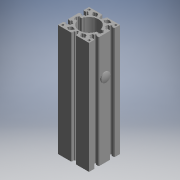
# Autodesk Inventor part: SLZ_63_Profil#_2871
Saved by Autodesk Inventor 2017.3 (Build 213256000, 256)
## iProperties
Part Number: SLZ_63_Profil#_2871
Material: Generic
Catalog Web Link: www.cadenas.de
Description: Profil Elektrozylinder SLZ 63-Control-Tec
Vendor: ROSEKRIEGER
Document SubType Name: Modeling
Designer: partserver
Manufacturer: ROSEKRIEGER
Mass: 785.447 g
Surface Area: 2909.04 cm^2
Volume: 785.447 cm^3
Density: 1 g/cm^3
Appearance: PSOLRGB-191-191-191
Category: PARTsolutions
Company: ROSEKRIEGER
Title: SLZ_63_Profil#_2871
Author: Cadenas PARTsolutions
Comments: Control-Tec
PSOL_IDENT_0: {$CADENAS_DATA\23d-libs\rose_krieger\linearkomponenten\pool_lineartechnik\_hubsaeule_zyliinder\elekt
PSOL_IDENT_1: rozylinder\elekzyl_slz63\parts\slz63_plfl_profil.prj},202 {VTYP=3D},{NB=SLZ_63_Profil#_2871},{LINA=S
PSOL_IDENT_2: LZ_63_Profil#_2871},{NN=Profil Elektrozylinder SLZ 63},{DATE=02.12.2020 11:16:24},{GEOMDATE=01.03.20
PSOL_IDENT_3: 17 09:52:29},{VERSION=},{LINEID=810},{WBVAR=},{WBNUMERIC=}  {NB=SLZ_63_Profil#_2871},{LINA=SLZ_63_Pr
PSOL_IDENT_4: ofil#_2871},{KT=DUMMY},{IDNR=},{CODE=TQ3},{ARTIKEL=Elektrozylinder },{TYPE=SLZ 63 Tr P PL},{BEST=SLZ
PSOL_IDENT_5: _63_Profil},{VARIANTE=PL},{SPINDEL=Tr 28x10},{SPINDELCODE=1.000},{SCHUTZARTVIS=IP54},{SCHUTZART=1},{
PSOL_IDENT_6: HUB1=0,[0:200]},{HUB2=200},{L1=287},{HINWEINBAUX=Hub + 274.5 mm},{DUMMYDURCH=10.000},{DUMMYLAENG=20.
PSOL_IDENT_7: 000},{HILFEHUB=105},{LAENDOPPROFIL=184.500},{RF=1.000},{GRUNDKOE=274.500},{XX=95.000},{A=100},{B=80}
PSOL_IDENT_8: ,{C=100},{D=125},{E=238},{F=40},{G=M16x1.5},{H=104},{K=125},{L=105},{M=48},{N=56.5},{O=86},{P=18.5},
PSOL_IDENT_9: {PPATH=sbl_lz70p_plfl.prj}
NB: SLZ_63_Profil#_2871
NN: Profil Elektrozylinder SLZ 63
NT: Control-Tec
NBSYN: $BEST.#_$L1.$SCHUTZART.
LINA: SLZ_63_Profil#_2871
CATALOG: RK Rose+Krieger
ARTIKEL: Elektrozylinder
TYPE: SLZ 63 Tr P PL
BEST: SLZ_63_Profil
SPINDEL: Tr 28x10
SPINDELCODE: 1
SCHUTZARTVIS: IP54
SCHUTZART: 1
HUB1: 0,[0:200]
HUB2: 200
L1: 287
HINWEINBAUX: Hub + 274.5 mm
DUMMYDURCH: 10
DUMMYLAENG: 20
HILFEHUB: 105
LAENDOPPROFIL: 184.5
RF: 1
GRUNDKOE: 274.5
XX: 95
A: 100
B: 80
C: 100
D: 125
E: 238
F: 40
G: M16x1.5
H: 104
K: 125
L: 105
M: 48
N: 56.5
O: 86
P: 18.5
SUPPLIER: ROSEKRIEGER
ARTICLENO: SLZ_63_Profil#_2871
BOMINFO: SLZ_63_Profil#_2871
CREATOR: CADENAS GmbH
Autodesk Inventor part; units mm, degrees
sketch "Sketch_1" plane through (0, 0, 0) normal (0, 0, 1) x (1, 0, 0)
  line L0 (-40, -26.375) -> (-40, -40)
  line L1 (-40, -40) -> (-6.3, -40)
  arc A0 (-6.3, -40) -> (-6.1, -39.8) centre (-6.3, -39.8) ccw
  line L2 (-6.1, -39.8) -> (-6.1, -38.7)
  arc A1 (-5.9, -38.5) -> (-6.1, -38.7) centre (-5.9, -38.7) ccw
  line L3 (-5.9, -38.5) -> (-5.3, -38.5)
  arc A2 (-5.3, -38.5) -> (-5.1, -38.3) centre (-5.3, -38.3) ccw
  line L4 (-5.1, -38.3) -> (-5.1, -33.2)
  arc A3 (-4.9, -33) -> (-5.1, -33.2) centre (-4.9, -33.2) ccw
  line L5 (-4.9, -33) -> (-2.95, -33)
  arc A4 (-2.95, -33) -> (-2.75, -32.8) centre (-2.95, -32.8) ccw
  line L6 (-2.75, -32.8) -> (-2.75, -28.6)
  arc A5 (-2.55, -28.4) -> (-2.75, -28.6) centre (-2.55, -28.6) ccw
  line L7 (-2.55, -28.4) -> (2.55, -28.4)
  arc A6 (2.75, -28.6) -> (2.55, -28.4) centre (2.55, -28.6) ccw
  line L8 (2.75, -28.6) -> (2.75, -32.8)
  arc A7 (2.75, -32.8) -> (2.95, -33) centre (2.95, -32.8) ccw
  line L9 (2.95, -33) -> (4.9, -33)
  arc A8 (5.1, -33.2) -> (4.9, -33) centre (4.9, -33.2) ccw
  line L10 (5.1, -33.2) -> (5.1, -38.3)
  arc A9 (5.1, -38.3) -> (5.3, -38.5) centre (5.3, -38.3) ccw
  line L11 (5.3, -38.5) -> (5.9, -38.5)
  arc A10 (6.1, -38.7) -> (5.9, -38.5) centre (5.9, -38.7) ccw
  line L12 (6.1, -38.7) -> (6.1, -39.8)
  arc A11 (6.1, -39.8) -> (6.3, -40) centre (6.3, -39.8) ccw
  line L13 (6.3, -40) -> (40, -40)
  line L14 (40, -40) -> (40, -26.375)
  arc A12 (40, -26.375) -> (39.7, -26.075) centre (39.7, -26.375) ccw
  line L15 (39.7, -26.075) -> (38.7, -26.075)
  arc A13 (38.5, -25.875) -> (38.7, -26.075) centre (38.7, -25.875) ccw
  line L16 (38.5, -25.875) -> (38.5, -25.4)
  arc A14 (38.5, -25.4) -> (38.2, -25.1) centre (38.2, -25.4) ccw
  line L17 (38.2, -25.1) -> (33.2, -25.1)
  arc A15 (33.2, -25.1) -> (33, -25.3) centre (33.2, -25.3) ccw
  line L18 (33, -25.3) -> (33, -27.55)
  arc A16 (32.8, -27.75) -> (33, -27.55) centre (32.8, -27.55) ccw
  line L19 (32.8, -27.75) -> (29.8328, -27.75)
  arc A17 (29.6914, -27.6914) -> (29.8328, -27.75) centre (29.8328, -27.55) ccw
  line L20 (29.6914, -27.6914) -> (28.5586, -26.5586)
  arc A18 (28.5, -26.4172) -> (28.5586, -26.5586) centre (28.7, -26.4172) ccw
  line L21 (28.5, -26.4172) -> (28.5, -24.45)
  arc A19 (28.5, -24.45) -> (28.3, -24.25) centre (28.3, -24.45) ccw
  line L22 (28.3, -24.25) -> (25, -24.25)
  arc A20 (24, -23.25) -> (25, -24.25) centre (25, -23.25) ccw
  line L23 (24, -23.25) -> (24, -20.3)
  arc A21 (24, -19.7) -> (24, -20.3) centre (24, -20) ccw
  line L24 (24, -19.7) -> (24, -16.75)
  arc A22 (25, -15.75) -> (24, -16.75) centre (25, -16.75) ccw
  line L25 (25, -15.75) -> (28.3, -15.75)
  arc A23 (28.3, -15.75) -> (28.5, -15.55) centre (28.3, -15.55) ccw
  line L26 (28.5, -15.55) -> (28.5, -13.5828)
  arc A24 (28.5586, -13.4414) -> (28.5, -13.5828) centre (28.7, -13.5828) ccw
  line L27 (28.5586, -13.4414) -> (29.6914, -12.3086)
  arc A25 (29.8328, -12.25) -> (29.6914, -12.3086) centre (29.8328, -12.45) ccw
  line L28 (29.8328, -12.25) -> (32.8, -12.25)
  arc A26 (33, -12.45) -> (32.8, -12.25) centre (32.8, -12.45) ccw
  line L29 (33, -12.45) -> (33, -14.7)
  arc A27 (33, -14.7) -> (33.2, -14.9) centre (33.2, -14.7) ccw
  line L30 (33.2, -14.9) -> (38.2, -14.9)
  arc A28 (38.2, -14.9) -> (38.5, -14.6) centre (38.2, -14.6) ccw
  line L31 (38.5, -14.6) -> (38.5, -14.125)
  arc A29 (38.7, -13.925) -> (38.5, -14.125) centre (38.7, -14.125) ccw
  line L32 (38.7, -13.925) -> (39.7, -13.925)
  arc A30 (39.7, -13.925) -> (40, -13.625) centre (39.7, -13.625) ccw
  line L33 (40, -13.625) -> (40, 13.625)
  arc A31 (40, 13.625) -> (39.7, 13.925) centre (39.7, 13.625) ccw
  line L34 (39.7, 13.925) -> (38.7, 13.925)
  arc A32 (38.5, 14.125) -> (38.7, 13.925) centre (38.7, 14.125) ccw
  line L35 (38.5, 14.125) -> (38.5, 14.6)
  arc A33 (38.5, 14.6) -> (38.2, 14.9) centre (38.2, 14.6) ccw
  line L36 (38.2, 14.9) -> (33.2, 14.9)
  arc A34 (33.2, 14.9) -> (33, 14.7) centre (33.2, 14.7) ccw
  line L37 (33, 14.7) -> (33, 12.45)
  arc A35 (32.8, 12.25) -> (33, 12.45) centre (32.8, 12.45) ccw
  line L38 (32.8, 12.25) -> (29.8328, 12.25)
  arc A36 (29.6914, 12.3086) -> (29.8328, 12.25) centre (29.8328, 12.45) ccw
  line L39 (29.6914, 12.3086) -> (28.5586, 13.4414)
  arc A37 (28.5, 13.5828) -> (28.5586, 13.4414) centre (28.7, 13.5828) ccw
  line L40 (28.5, 13.5828) -> (28.5, 15.55)
  arc A38 (28.5, 15.55) -> (28.3, 15.75) centre (28.3, 15.55) ccw
  line L41 (28.3, 15.75) -> (25, 15.75)
  arc A39 (24, 16.75) -> (25, 15.75) centre (25, 16.75) ccw
  line L42 (24, 16.75) -> (24, 19.7)
  arc A40 (24, 20.3) -> (24, 19.7) centre (24, 20) ccw
  line L43 (24, 20.3) -> (24, 23.25)
  arc A41 (25, 24.25) -> (24, 23.25) centre (25, 23.25) ccw
  line L44 (25, 24.25) -> (28.3, 24.25)
  arc A42 (28.3, 24.25) -> (28.5, 24.45) centre (28.3, 24.45) ccw
  line L45 (28.5, 24.45) -> (28.5, 26.4172)
  arc A43 (28.5586, 26.5586) -> (28.5, 26.4172) centre (28.7, 26.4172) ccw
  line L46 (28.5586, 26.5586) -> (29.6914, 27.6914)
  arc A44 (29.8328, 27.75) -> (29.6914, 27.6914) centre (29.8328, 27.55) ccw
  line L47 (29.8328, 27.75) -> (32.8, 27.75)
  arc A45 (33, 27.55) -> (32.8, 27.75) centre (32.8, 27.55) ccw
  line L48 (33, 27.55) -> (33, 25.3)
  arc A46 (33, 25.3) -> (33.2, 25.1) centre (33.2, 25.3) ccw
  line L49 (33.2, 25.1) -> (38.2, 25.1)
  arc A47 (38.2, 25.1) -> (38.5, 25.4) centre (38.2, 25.4) ccw
  line L50 (38.5, 25.4) -> (38.5, 25.875)
  arc A48 (38.7, 26.075) -> (38.5, 25.875) centre (38.7, 25.875) ccw
  line L51 (38.7, 26.075) -> (39.7, 26.075)
  arc A49 (39.7, 26.075) -> (40, 26.375) centre (39.7, 26.375) ccw
  line L52 (40, 26.375) -> (40, 40)
  line L53 (40, 40) -> (6.3, 40)
  arc A50 (6.3, 40) -> (6.1, 39.8) centre (6.3, 39.8) ccw
  line L54 (6.1, 39.8) -> (6.1, 38.7)
  arc A51 (5.9, 38.5) -> (6.1, 38.7) centre (5.9, 38.7) ccw
  line L55 (5.9, 38.5) -> (5.3, 38.5)
  arc A52 (5.3, 38.5) -> (5.1, 38.3) centre (5.3, 38.3) ccw
  line L56 (5.1, 38.3) -> (5.1, 33.2)
  arc A53 (4.9, 33) -> (5.1, 33.2) centre (4.9, 33.2) ccw
  line L57 (4.9, 33) -> (2.95, 33)
  arc A54 (2.95, 33) -> (2.75, 32.8) centre (2.95, 32.8) ccw
  line L58 (2.75, 32.8) -> (2.75, 28.6)
  arc A55 (2.55, 28.4) -> (2.75, 28.6) centre (2.55, 28.6) ccw
  line L59 (2.55, 28.4) -> (-2.55, 28.4)
  arc A56 (-2.75, 28.6) -> (-2.55, 28.4) centre (-2.55, 28.6) ccw
  line L60 (-2.75, 28.6) -> (-2.75, 32.8)
  arc A57 (-2.75, 32.8) -> (-2.95, 33) centre (-2.95, 32.8) ccw
  line L61 (-2.95, 33) -> (-4.9, 33)
  arc A58 (-5.1, 33.2) -> (-4.9, 33) centre (-4.9, 33.2) ccw
  line L62 (-5.1, 33.2) -> (-5.1, 38.3)
  arc A59 (-5.1, 38.3) -> (-5.3, 38.5) centre (-5.3, 38.3) ccw
  line L63 (-5.3, 38.5) -> (-5.9, 38.5)
  arc A60 (-6.1, 38.7) -> (-5.9, 38.5) centre (-5.9, 38.7) ccw
  line L64 (-6.1, 38.7) -> (-6.1, 39.8)
  arc A61 (-6.1, 39.8) -> (-6.3, 40) centre (-6.3, 39.8) ccw
  line L65 (-6.3, 40) -> (-40, 40)
  line L66 (-40, 40) -> (-40, 26.375)
  arc A62 (-40, 26.375) -> (-39.7, 26.075) centre (-39.7, 26.375) ccw
  line L67 (-39.7, 26.075) -> (-38.7, 26.075)
  arc A63 (-38.5, 25.875) -> (-38.7, 26.075) centre (-38.7, 25.875) ccw
  line L68 (-38.5, 25.875) -> (-38.5, 25.4)
  arc A64 (-38.5, 25.4) -> (-38.2, 25.1) centre (-38.2, 25.4) ccw
  line L69 (-38.2, 25.1) -> (-33.2, 25.1)
  arc A65 (-33.2, 25.1) -> (-33, 25.3) centre (-33.2, 25.3) ccw
  line L70 (-33, 25.3) -> (-33, 27.55)
  arc A66 (-32.8, 27.75) -> (-33, 27.55) centre (-32.8, 27.55) ccw
  line L71 (-32.8, 27.75) -> (-29.8328, 27.75)
  arc A67 (-29.6914, 27.6914) -> (-29.8328, 27.75) centre (-29.8328, 27.55) ccw
  line L72 (-29.6914, 27.6914) -> (-28.5586, 26.5586)
  arc A68 (-28.5, 26.4172) -> (-28.5586, 26.5586) centre (-28.7, 26.4172) ccw
  line L73 (-28.5, 26.4172) -> (-28.5, 24.45)
  arc A69 (-28.5, 24.45) -> (-28.3, 24.25) centre (-28.3, 24.45) ccw
  line L74 (-28.3, 24.25) -> (-25, 24.25)
  arc A70 (-24, 23.25) -> (-25, 24.25) centre (-25, 23.25) ccw
  line L75 (-24, 23.25) -> (-24, 20.3)
  arc A71 (-24, 19.7) -> (-24, 20.3) centre (-24, 20) ccw
  line L76 (-24, 19.7) -> (-24, 16.75)
  arc A72 (-25, 15.75) -> (-24, 16.75) centre (-25, 16.75) ccw
  line L77 (-25, 15.75) -> (-28.3, 15.75)
  arc A73 (-28.3, 15.75) -> (-28.5, 15.55) centre (-28.3, 15.55) ccw
  line L78 (-28.5, 15.55) -> (-28.5, 13.5828)
  arc A74 (-28.5586, 13.4414) -> (-28.5, 13.5828) centre (-28.7, 13.5828) ccw
  line L79 (-28.5586, 13.4414) -> (-29.6914, 12.3086)
  arc A75 (-29.8328, 12.25) -> (-29.6914, 12.3086) centre (-29.8328, 12.45) ccw
  line L80 (-29.8328, 12.25) -> (-32.8, 12.25)
  arc A76 (-33, 12.45) -> (-32.8, 12.25) centre (-32.8, 12.45) ccw
  line L81 (-33, 12.45) -> (-33, 14.7)
  arc A77 (-33, 14.7) -> (-33.2, 14.9) centre (-33.2, 14.7) ccw
  line L82 (-33.2, 14.9) -> (-38.2, 14.9)
  arc A78 (-38.2, 14.9) -> (-38.5, 14.6) centre (-38.2, 14.6) ccw
  line L83 (-38.5, 14.6) -> (-38.5, 14.125)
  arc A79 (-38.7, 13.925) -> (-38.5, 14.125) centre (-38.7, 14.125) ccw
  line L84 (-38.7, 13.925) -> (-39.7, 13.925)
  arc A80 (-39.7, 13.925) -> (-40, 13.625) centre (-39.7, 13.625) ccw
  line L85 (-40, 13.625) -> (-40, -13.625)
  arc A81 (-40, -13.625) -> (-39.7, -13.925) centre (-39.7, -13.625) ccw
  line L86 (-39.7, -13.925) -> (-38.7, -13.925)
  arc A82 (-38.5, -14.125) -> (-38.7, -13.925) centre (-38.7, -14.125) ccw
  line L87 (-38.5, -14.125) -> (-38.5, -14.6)
  arc A83 (-38.5, -14.6) -> (-38.2, -14.9) centre (-38.2, -14.6) ccw
  line L88 (-38.2, -14.9) -> (-33.2, -14.9)
  arc A84 (-33.2, -14.9) -> (-33, -14.7) centre (-33.2, -14.7) ccw
  line L89 (-33, -14.7) -> (-33, -12.45)
  arc A85 (-32.8, -12.25) -> (-33, -12.45) centre (-32.8, -12.45) ccw
  line L90 (-32.8, -12.25) -> (-29.8328, -12.25)
  arc A86 (-29.6914, -12.3086) -> (-29.8328, -12.25) centre (-29.8328, -12.45) ccw
  line L91 (-29.6914, -12.3086) -> (-28.5586, -13.4414)
  arc A87 (-28.5, -13.5828) -> (-28.5586, -13.4414) centre (-28.7, -13.5828) ccw
  line L92 (-28.5, -13.5828) -> (-28.5, -15.55)
  arc A88 (-28.5, -15.55) -> (-28.3, -15.75) centre (-28.3, -15.55) ccw
  line L93 (-28.3, -15.75) -> (-25, -15.75)
  arc A89 (-24, -16.75) -> (-25, -15.75) centre (-25, -16.75) ccw
  line L94 (-24, -16.75) -> (-24, -19.7)
  arc A90 (-24, -20.3) -> (-24, -19.7) centre (-24, -20) ccw
  line L95 (-24, -20.3) -> (-24, -23.25)
  arc A91 (-25, -24.25) -> (-24, -23.25) centre (-25, -23.25) ccw
  line L96 (-25, -24.25) -> (-28.3, -24.25)
  arc A92 (-28.3, -24.25) -> (-28.5, -24.45) centre (-28.3, -24.45) ccw
  line L97 (-28.5, -24.45) -> (-28.5, -26.4172)
  arc A93 (-28.5586, -26.5586) -> (-28.5, -26.4172) centre (-28.7, -26.4172) ccw
  line L98 (-28.5586, -26.5586) -> (-29.6914, -27.6914)
  arc A94 (-29.8328, -27.75) -> (-29.6914, -27.6914) centre (-29.8328, -27.55) ccw
  line L99 (-29.8328, -27.75) -> (-32.8, -27.75)
  arc A95 (-33, -27.55) -> (-32.8, -27.75) centre (-32.8, -27.55) ccw
  line L100 (-33, -27.55) -> (-33, -25.3)
  arc A96 (-33, -25.3) -> (-33.2, -25.1) centre (-33.2, -25.3) ccw
  line L101 (-33.2, -25.1) -> (-38.2, -25.1)
  arc A97 (-38.2, -25.1) -> (-38.5, -25.4) centre (-38.2, -25.4) ccw
  line L102 (-38.5, -25.4) -> (-38.5, -25.875)
  arc A98 (-38.7, -26.075) -> (-38.5, -25.875) centre (-38.7, -25.875) ccw
  line L103 (-38.7, -26.075) -> (-39.7, -26.075)
  arc A99 (-39.7, -26.075) -> (-40, -26.375) centre (-39.7, -26.375) ccw
  arc A100 (31.6024, 35.3468) -> (31.6024, 32.6532) centre (34, 34) ccw
  arc A101 (31.6024, 32.6532) -> (32.6532, 31.6024) centre (32.0555, 32.0555) ccw
  arc A102 (32.6532, 31.6024) -> (35.3468, 31.6024) centre (34, 34) ccw
  arc A103 (35.3468, 31.6024) -> (36.3976, 32.6532) centre (35.9445, 32.0555) ccw
  arc A104 (36.3976, 32.6532) -> (36.3976, 35.3468) centre (34, 34) ccw
  arc A105 (36.3976, 35.3468) -> (35.3468, 36.3976) centre (35.9445, 35.9445) ccw
  arc A106 (35.3468, 36.3976) -> (32.6532, 36.3976) centre (34, 34) ccw
  arc A107 (32.6532, 36.3976) -> (31.6024, 35.3468) centre (32.0555, 35.9445) ccw
  arc A108 (31.6024, -32.6532) -> (31.6024, -35.3468) centre (34, -34) ccw
  arc A109 (31.6024, -35.3468) -> (32.6532, -36.3976) centre (32.0555, -35.9445) ccw
  arc A110 (32.6532, -36.3976) -> (35.3468, -36.3976) centre (34, -34) ccw
  arc A111 (35.3468, -36.3976) -> (36.3976, -35.3468) centre (35.9445, -35.9445) ccw
  arc A112 (36.3976, -35.3468) -> (36.3976, -32.6532) centre (34, -34) ccw
  arc A113 (36.3976, -32.6532) -> (35.3468, -31.6024) centre (35.9445, -32.0555) ccw
  arc A114 (35.3468, -31.6024) -> (32.6532, -31.6024) centre (34, -34) ccw
  arc A115 (32.6532, -31.6024) -> (31.6024, -32.6532) centre (32.0555, -32.0555) ccw
  arc A116 (10.3501, 31.0384) -> (11.6966, 27.3389) centre (10.6907, 29.0676) ccw
  arc A117 (11.6966, 27.3389) -> (21.6499, 30.9616) centre (16, 31) ccw
  arc A118 (21.6499, 30.9616) -> (20.3034, 34.6611) centre (21.3093, 32.9324) ccw
  arc A119 (20.3034, 34.6611) -> (10.3501, 31.0384) centre (16, 31) ccw
  arc A120 (11.6966, -27.3389) -> (10.3501, -31.0384) centre (10.6907, -29.0676) ccw
  arc A121 (10.3501, -31.0384) -> (20.3034, -34.6611) centre (16, -31) ccw
  arc A122 (20.3034, -34.6611) -> (21.6499, -30.9616) centre (21.3093, -32.9324) ccw
  arc A123 (21.6499, -30.9616) -> (11.6966, -27.3389) centre (16, -31) ccw
  arc A124 (-21.6499, -30.9616) -> (-20.3034, -34.6611) centre (-21.3093, -32.9324) ccw
  arc A125 (-20.3034, -34.6611) -> (-10.3501, -31.0384) centre (-16, -31) ccw
  arc A126 (-10.3501, -31.0384) -> (-11.6966, -27.3389) centre (-10.6907, -29.0676) ccw
  arc A127 (-11.6966, -27.3389) -> (-21.6499, -30.9616) centre (-16, -31) ccw
  arc A128 (-20.3034, 34.6611) -> (-21.6499, 30.9616) centre (-21.3093, 32.9324) ccw
  arc A129 (-21.6499, 30.9616) -> (-11.6966, 27.3389) centre (-16, 31) ccw
  arc A130 (-11.6966, 27.3389) -> (-10.3501, 31.0384) centre (-10.6907, 29.0676) ccw
  arc A131 (-10.3501, 31.0384) -> (-20.3034, 34.6611) centre (-16, 31) ccw
  line L104 (-35, 1.95) -> (-35, -1.95)
  arc A132 (-35, -1.95) -> (-34.8, -2.15) centre (-34.8, -1.95) ccw
  line L105 (-34.8, -2.15) -> (-33.7, -2.15)
  arc A133 (-33.5, -2.35) -> (-33.7, -2.15) centre (-33.7, -2.35) ccw
  line L106 (-33.5, -2.35) -> (-33.5, -4.95)
  arc A134 (-33.5, -4.95) -> (-33.3, -5.15) centre (-33.3, -4.95) ccw
  line L107 (-33.3, -5.15) -> (-31.7, -5.15)
  arc A135 (-31.5, -5.35) -> (-31.7, -5.15) centre (-31.7, -5.35) ccw
  line L108 (-31.5, -5.35) -> (-31.5, -7.1)
  arc A136 (-31.5, -7.1) -> (-31.3, -7.3) centre (-31.3, -7.1) ccw
  line L109 (-31.3, -7.3) -> (-30, -7.3)
  arc A137 (-30, -7.3) -> (-29.8, -7.1) centre (-30, -7.1) ccw
  line L110 (-29.8, -7.1) -> (-29.8, -5.3)
  arc A138 (-29.6, -5.1) -> (-29.8, -5.3) centre (-29.6, -5.3) ccw
  line L111 (-29.6, -5.1) -> (-29.4, -5.1)
  arc A139 (-29.2, -5.3) -> (-29.4, -5.1) centre (-29.4, -5.3) ccw
  arc A140 (-29.2, -5.3) -> (-29, -5.5) centre (-29, -5.3) ccw
  line L112 (-29, -5.5) -> (-24.5469, -5.5)
  arc A141 (-24.3521, -5.6548) -> (-24.5469, -5.5) centre (-24.5469, -5.7) ccw
  arc A142 (-24.3521, -5.6548) -> (-23.4523, -8.6598) centre (0, 0) ccw
  arc A143 (-23.4551, -8.8056) -> (-23.4523, -8.6598) centre (-23.6399, -8.7291) ccw
  line L113 (-23.4551, -8.8056) -> (-23.91, -9.9038)
  line L114 (-23.91, -9.9038) -> (-22.8118, -10.3588)
  arc A144 (-22.7066, -10.4599) -> (-22.8118, -10.3588) centre (-22.8883, -10.5435) ccw
  arc A145 (-22.7066, -10.4599) -> (-10.4599, -22.7066) centre (0, 0) ccw
  arc A146 (-10.3588, -22.8118) -> (-10.4599, -22.7066) centre (-10.5435, -22.8883) ccw
  line L115 (-10.3588, -22.8118) -> (-9.9804, -23.7252)
  arc A147 (-9.9804, -23.7252) -> (-9.7191, -23.8335) centre (-9.7956, -23.6487) ccw
  line L116 (-9.7191, -23.8335) -> (-8.8056, -23.4551)
  arc A148 (-8.6598, -23.4523) -> (-8.8056, -23.4551) centre (-8.7291, -23.6399) ccw
  arc A149 (-8.6598, -23.4523) -> (8.6598, -23.4523) centre (0, 0) ccw
  arc A150 (8.8056, -23.4551) -> (8.6598, -23.4523) centre (8.7291, -23.6399) ccw
  line L117 (8.8056, -23.4551) -> (9.7191, -23.8335)
  arc A151 (9.7191, -23.8335) -> (9.9804, -23.7252) centre (9.7956, -23.6487) ccw
  line L118 (9.9804, -23.7252) -> (10.3588, -22.8118)
  arc A152 (10.4599, -22.7066) -> (10.3588, -22.8118) centre (10.5435, -22.8883) ccw
  arc A153 (10.4599, -22.7066) -> (22.7066, -10.4599) centre (0, 0) ccw
  arc A154 (22.8118, -10.3588) -> (22.7066, -10.4599) centre (22.8883, -10.5435) ccw
  line L119 (22.8118, -10.3588) -> (23.91, -9.9038)
  line L120 (23.91, -9.9038) -> (23.4551, -8.8056)
  arc A155 (23.4523, -8.6598) -> (23.4551, -8.8056) centre (23.6399, -8.7291) ccw
  arc A156 (23.4523, -8.6598) -> (24.3521, -5.6548) centre (0, 0) ccw
  arc A157 (24.5469, -5.5) -> (24.3521, -5.6548) centre (24.5469, -5.7) ccw
  line L121 (24.5469, -5.5) -> (29, -5.5)
  arc A158 (29, -5.5) -> (29.2, -5.3) centre (29, -5.3) ccw
  arc A159 (29.4, -5.1) -> (29.2, -5.3) centre (29.4, -5.3) ccw
  line L122 (29.4, -5.1) -> (29.6, -5.1)
  arc A160 (29.8, -5.3) -> (29.6, -5.1) centre (29.6, -5.3) ccw
  line L123 (29.8, -5.3) -> (29.8, -7.1)
  arc A161 (29.8, -7.1) -> (30, -7.3) centre (30, -7.1) ccw
  line L124 (30, -7.3) -> (31.3, -7.3)
  arc A162 (31.3, -7.3) -> (31.5, -7.1) centre (31.3, -7.1) ccw
  line L125 (31.5, -7.1) -> (31.5, -5.35)
  arc A163 (31.7, -5.15) -> (31.5, -5.35) centre (31.7, -5.35) ccw
  line L126 (31.7, -5.15) -> (33.3, -5.15)
  arc A164 (33.3, -5.15) -> (33.5, -4.95) centre (33.3, -4.95) ccw
  line L127 (33.5, -4.95) -> (33.5, -2.35)
  arc A165 (33.7, -2.15) -> (33.5, -2.35) centre (33.7, -2.35) ccw
  line L128 (33.7, -2.15) -> (34.8, -2.15)
  arc A166 (34.8, -2.15) -> (35, -1.95) centre (34.8, -1.95) ccw
  line L129 (35, -1.95) -> (35, 1.95)
  arc A167 (35, 1.95) -> (34.8, 2.15) centre (34.8, 1.95) ccw
  line L130 (34.8, 2.15) -> (33.7, 2.15)
  arc A168 (33.5, 2.35) -> (33.7, 2.15) centre (33.7, 2.35) ccw
  line L131 (33.5, 2.35) -> (33.5, 4.95)
  arc A169 (33.5, 4.95) -> (33.3, 5.15) centre (33.3, 4.95) ccw
  line L132 (33.3, 5.15) -> (31.7, 5.15)
  arc A170 (31.5, 5.35) -> (31.7, 5.15) centre (31.7, 5.35) ccw
  line L133 (31.5, 5.35) -> (31.5, 7.1)
  arc A171 (31.5, 7.1) -> (31.3, 7.3) centre (31.3, 7.1) ccw
  line L134 (31.3, 7.3) -> (30, 7.3)
  arc A172 (30, 7.3) -> (29.8, 7.1) centre (30, 7.1) ccw
  line L135 (29.8, 7.1) -> (29.8, 5.3)
  arc A173 (29.6, 5.1) -> (29.8, 5.3) centre (29.6, 5.3) ccw
  line L136 (29.6, 5.1) -> (29.4, 5.1)
  arc A174 (29.2, 5.3) -> (29.4, 5.1) centre (29.4, 5.3) ccw
  arc A175 (29.2, 5.3) -> (29, 5.5) centre (29, 5.3) ccw
  line L137 (29, 5.5) -> (24.5469, 5.5)
  arc A176 (24.3521, 5.6548) -> (24.5469, 5.5) centre (24.5469, 5.7) ccw
  arc A177 (24.3521, 5.6548) -> (23.4523, 8.6598) centre (0, 0) ccw
  arc A178 (23.4551, 8.8056) -> (23.4523, 8.6598) centre (23.6399, 8.7291) ccw
  line L138 (23.4551, 8.8056) -> (23.91, 9.9038)
  line L139 (23.91, 9.9038) -> (22.8118, 10.3588)
  arc A179 (22.7066, 10.4599) -> (22.8118, 10.3588) centre (22.8883, 10.5435) ccw
  arc A180 (22.7066, 10.4599) -> (10.4599, 22.7066) centre (0, 0) ccw
  arc A181 (10.3588, 22.8118) -> (10.4599, 22.7066) centre (10.5435, 22.8883) ccw
  line L140 (10.3588, 22.8118) -> (9.9804, 23.7252)
  arc A182 (9.9804, 23.7252) -> (9.7191, 23.8335) centre (9.7956, 23.6487) ccw
  line L141 (9.7191, 23.8335) -> (8.8056, 23.4551)
  arc A183 (8.6598, 23.4523) -> (8.8056, 23.4551) centre (8.7291, 23.6399) ccw
  arc A184 (8.6598, 23.4523) -> (-8.6598, 23.4523) centre (0, 0) ccw
  arc A185 (-8.8056, 23.4551) -> (-8.6598, 23.4523) centre (-8.7291, 23.6399) ccw
  line L142 (-8.8056, 23.4551) -> (-9.7191, 23.8335)
  arc A186 (-9.7191, 23.8335) -> (-9.9804, 23.7252) centre (-9.7956, 23.6487) ccw
  line L143 (-9.9804, 23.7252) -> (-10.3588, 22.8118)
  arc A187 (-10.4599, 22.7066) -> (-10.3588, 22.8118) centre (-10.5435, 22.8883) ccw
  arc A188 (-10.4599, 22.7066) -> (-22.7066, 10.4599) centre (0, 0) ccw
  arc A189 (-22.8118, 10.3588) -> (-22.7066, 10.4599) centre (-22.8883, 10.5435) ccw
  line L144 (-22.8118, 10.3588) -> (-23.91, 9.9038)
  line L145 (-23.91, 9.9038) -> (-23.4551, 8.8056)
  arc A190 (-23.4523, 8.6598) -> (-23.4551, 8.8056) centre (-23.6399, 8.7291) ccw
  arc A191 (-23.4523, 8.6598) -> (-24.3521, 5.6548) centre (0, 0) ccw
  arc A192 (-24.5469, 5.5) -> (-24.3521, 5.6548) centre (-24.5469, 5.7) ccw
  line L146 (-24.5469, 5.5) -> (-29, 5.5)
  arc A193 (-29, 5.5) -> (-29.2, 5.3) centre (-29, 5.3) ccw
  arc A194 (-29.4, 5.1) -> (-29.2, 5.3) centre (-29.4, 5.3) ccw
  line L147 (-29.4, 5.1) -> (-29.6, 5.1)
  arc A195 (-29.8, 5.3) -> (-29.6, 5.1) centre (-29.6, 5.3) ccw
  line L148 (-29.8, 5.3) -> (-29.8, 7.1)
  arc A196 (-29.8, 7.1) -> (-30, 7.3) centre (-30, 7.1) ccw
  line L149 (-30, 7.3) -> (-31.3, 7.3)
  arc A197 (-31.3, 7.3) -> (-31.5, 7.1) centre (-31.3, 7.1) ccw
  line L150 (-31.5, 7.1) -> (-31.5, 5.35)
  arc A198 (-31.7, 5.15) -> (-31.5, 5.35) centre (-31.7, 5.35) ccw
  line L151 (-31.7, 5.15) -> (-33.3, 5.15)
  arc A199 (-33.3, 5.15) -> (-33.5, 4.95) centre (-33.3, 4.95) ccw
  line L152 (-33.5, 4.95) -> (-33.5, 2.35)
  arc A200 (-33.7, 2.15) -> (-33.5, 2.35) centre (-33.7, 2.35) ccw
  line L153 (-33.7, 2.15) -> (-34.8, 2.15)
  arc A201 (-34.8, 2.15) -> (-35, 1.95) centre (-34.8, 1.95) ccw
  arc A202 (-36.3976, 35.3468) -> (-36.3976, 32.6532) centre (-34, 34) ccw
  arc A203 (-36.3976, 32.6532) -> (-35.3468, 31.6024) centre (-35.9445, 32.0555) ccw
  arc A204 (-35.3468, 31.6024) -> (-32.6532, 31.6024) centre (-34, 34) ccw
  arc A205 (-32.6532, 31.6024) -> (-31.6024, 32.6532) centre (-32.0555, 32.0555) ccw
  arc A206 (-31.6024, 32.6532) -> (-31.6024, 35.3468) centre (-34, 34) ccw
  arc A207 (-31.6024, 35.3468) -> (-32.6532, 36.3976) centre (-32.0555, 35.9445) ccw
  arc A208 (-32.6532, 36.3976) -> (-35.3468, 36.3976) centre (-34, 34) ccw
  arc A209 (-35.3468, 36.3976) -> (-36.3976, 35.3468) centre (-35.9445, 35.9445) ccw
  arc A210 (-36.3976, -32.6532) -> (-36.3976, -35.3468) centre (-34, -34) ccw
  arc A211 (-36.3976, -35.3468) -> (-35.3468, -36.3976) centre (-35.9445, -35.9445) ccw
  arc A212 (-35.3468, -36.3976) -> (-32.6532, -36.3976) centre (-34, -34) ccw
  arc A213 (-32.6532, -36.3976) -> (-31.6024, -35.3468) centre (-32.0555, -35.9445) ccw
  arc A214 (-31.6024, -35.3468) -> (-31.6024, -32.6532) centre (-34, -34) ccw
  arc A215 (-31.6024, -32.6532) -> (-32.6532, -31.6024) centre (-32.0555, -32.0555) ccw
  arc A216 (-32.6532, -31.6024) -> (-35.3468, -31.6024) centre (-34, -34) ccw
  arc A217 (-35.3468, -31.6024) -> (-36.3976, -32.6532) centre (-35.9445, -32.0555) ccw
  constraints: 436 point on circle, 308 end point, 218 centre point
extrude "Extrusion1" add sketch "Sketch_1" along normal blind 287
sketch "Sketch_2" plane through (0, 0, 0) normal (1, 0, 0) x (0, 0, -1)
  line L0 (-269, 0) -> (-269, 40)
  line L1 (-269, 40) -> (-266.9, 40)
  line L2 (-266.9, 40) -> (-266.9, 0)
  line L3 (-266.9, 0) -> (-269, 0)
  line L4 (-269, 0) -> (-269, 40)
  constraints: 10 end point
revolve "Revolution1" cut sketch "Sketch_2" angle 360 about axis through (0, 0, 269) along (0, -1, 0)
sketch "Sketch_6" plane through (0, 0, 0) normal (0, 1, 0) x (1, 0, 0)
  line L0 (-35.5, -95) -> (-45.0008, -95)
  arc A0 (-43.25, -83) -> (-45.0008, -95) centre (-3.0008, -95) ccw
  line L1 (-43.25, -83) -> (-41.5, -83)
  line L2 (-41.5, -83) -> (-41.5, -84.25)
  arc A1 (-40, -84.25) -> (-41.5, -84.25) centre (-40.75, -84.25) ccw
  line L3 (-40, -84.25) -> (-40, -85)
  line L4 (-40, -85) -> (-36.8, -85)
  line L5 (-36.8, -85) -> (-35.5, -85.7506)
  line L6 (-35.5, -85.7506) -> (-35.5, -95)
  line L7 (-35.5, -95) -> (-45.0008, -95)
  constraints: 16 end point, 4 point on circle, 2 centre point
revolve "Revolution2" add sketch "Sketch_6" angle 360 about axis through (-35.5, 0, 95) along (1, 0, 0)
ref_plane "ABDECKPROFIL1_XY" through (0, 40, 287) normal (0, 0, 1) x (1, 0, 0)
ref_plane "ABDECKPROFIL1_YZ" through (0, 40, 287) normal (1, 0, 0) x (0, 1, 0)
ref_plane "ABDECKPROFIL1_ZX" through (0, 40, 287) normal (0, 1, 0) x (0, 0, 1)
ref_plane "ABDECKPROFIL2_XY" through (40, 20, 287) normal (0, 0, 1) x (1, 0, 0)
ref_plane "ABDECKPROFIL2_YZ" through (40, 20, 287) normal (1, 0, 0) x (0, 1, 0)
ref_plane "ABDECKPROFIL2_ZX" through (40, 20, 287) normal (0, 1, 0) x (0, 0, 1)
ref_plane "ABDECKPROFIL3_XY" through (40, -20, 287) normal (0, 0, 1) x (1, 0, 0)
ref_plane "ABDECKPROFIL3_YZ" through (40, -20, 287) normal (1, 0, 0) x (0, 1, 0)
ref_plane "ABDECKPROFIL3_ZX" through (40, -20, 287) normal (0, 1, 0) x (0, 0, 1)
ref_plane "ABDECKPROFIL4_XY" through (0, -40, 287) normal (0, 0, 1) x (1, 0, 0)
ref_plane "ABDECKPROFIL4_YZ" through (0, -40, 287) normal (1, 0, 0) x (0, 1, 0)
ref_plane "ABDECKPROFIL4_ZX" through (0, -40, 287) normal (0, 1, 0) x (0, 0, 1)
ref_plane "ABDECKPROFIL5_XY" through (-40, -20, 287) normal (0, 0, 1) x (1, 0, 0)
ref_plane "ABDECKPROFIL5_YZ" through (-40, -20, 287) normal (1, 0, 0) x (0, 1, 0)
ref_plane "ABDECKPROFIL5_ZX" through (-40, -20, 287) normal (0, 1, 0) x (0, 0, 1)
ref_plane "ABDECKPROFIL6_XY" through (-40, 20, 287) normal (0, 0, 1) x (1, 0, 0)
ref_plane "ABDECKPROFIL6_YZ" through (-40, 20, 287) normal (1, 0, 0) x (0, 1, 0)
ref_plane "ABDECKPROFIL6_ZX" through (-40, 20, 287) normal (0, 1, 0) x (0, 0, 1)
ref_plane "ANTRIEBGEHAEUSE_XY" through (0, 0, 0) normal (0, 0, 1) x (1, 0, 0)
ref_plane "ANTRIEBGEHAEUSE_YZ" through (0, 0, 0) normal (1, 0, 0) x (0, 1, 0)
ref_plane "ANTRIEBGEHAEUSE_ZX" through (0, 0, 0) normal (0, 1, 0) x (0, 0, 1)
ref_plane "DPL2_XY" through (0, 0, 95) normal (1, 0, 0) x (0, 0, -1)
ref_plane "DPL2_YZ" through (0, 0, 95) normal (0, 0, -1) x (0, 1, 0)
ref_plane "DPL2_ZX" through (0, 0, 95) normal (0, 1, 0) x (1, 0, 0)
ref_plane "DPLHUB2_XY" through (0, 0, 205) normal (1, 0, 0) x (0, 0, -1)
ref_plane "DPLHUB2_YZ" through (0, 0, 205) normal (0, 0, -1) x (0, 1, 0)
ref_plane "DPLHUB2_ZX" through (0, 0, 205) normal (0, 1, 0) x (1, 0, 0)
ref_plane "PROFIL_XY" through (0, 0, 287) normal (0, 0, -1) x (1, 0, 0)
ref_plane "PROFIL_YZ" through (0, 0, 287) normal (1, 0, 0) x (0, -1, 0)
ref_plane "PROFIL_ZX" through (0, 0, 287) normal (0, -1, 0) x (0, 0, -1)
body "Solid1"
